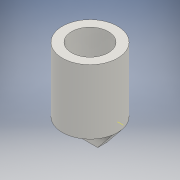
# Autodesk Inventor part: стакан_v2
Saved by Autodesk Inventor 2017.3 (Build 213256000, 256)
## iProperties
Part Number: стакан_v2
Material: Сталь
Document SubType Name: Modeling
Designer: Alexnav
Density: 7.85 g/cm^3
Appearance: По умолчанию
Mass: 1042.58 g
Surface Area: 290.439 cm^2
Volume: 132.812 cm^3
Author: Alexnav
Autodesk Inventor part; units mm, degrees
ref_plane "YZ Plane" through (0, 0, 0) normal (1, 0, 0) x (0, 1, 0)
ref_plane "XZ Plane" through (0, 0, 0) normal (0, 1, 0) x (-1, 0, 0)
ref_plane "XY Plane" through (0, 0, 0) normal (0, 0, 1) x (1, 0, 0)
sketch "Эскиз1" plane through (0, 0, 0) normal (0, 0, 1) x (1, 0, 0)
  circle A0 centre (0, 0) radius 20
  circle A1 centre (0, 0) radius 30
  dimension "d0" = 40
  dimension "d1" = 10
  constraints: 2 centre point, 2 coincident
  measures "d0" diameter of A0
  measures "d1" radial gap between concentric circles of A1 A0
extrude "Выдавливание1" add sketch "Эскиз1" along normal blind 60
sketch "Эскиз2" plane through (0, 0, 0) normal (0, 0, -1) x (-1, 0, 0)
  circle A0 centre (0, 0) radius 30 projected
extrude "Выдавливание2" add sketch "Эскиз2" along normal blind 10
sketch "Эскиз3" plane through (0, 0, -10) normal (0, 0, -1) x (-1, 0, 0)
  circle A0 centre (0, 0) radius 30 projected
  line L0 (-29.5804, 5) -> (29.5804, 5)
  line L1 (29.5804, -5) -> (-29.5804, -5)
  line L2 (42, 0) -> (-42, 0) projected
  dimension "d7" = 10
  constraints: 4 end point, 4 point on circle, 1 horizontal, 1 parallel, 1 other
  measures "d7" distance between parallel lines of L1 L0
extrude "Выдавливание3" add sketch "Эскиз3" along normal blind 20 contours L2 A0 L0 | A0 L1 L2
sketch "Эскиз4" plane through (-29.5804, 5, -10) normal (0, 1, 0) x (1, 0, 0)
  line L0 (59.1608, 0) -> (0, 0) projected
  line L1 (59.1608, 0) -> (59.1608, 20) projected
  line L2 (0, 20) -> (59.1608, 20) projected
  line L3 (0, 0) -> (0, 20) projected
  line L4 (59.1608, 0) -> (59.1608, 20) projected
  line L5 (0, 0) -> (59.1608, 0) projected
  line L6 (0, 0) -> (0, 20) projected
  line L7 (0, 20) -> (59.1608, 20) projected
  circle A0 centre (29.5804, 10) radius 5
  point P0 (29.5804, -10)
  dimension "d11" = 10
  constraints: 1 centre point
  measures "d11" diameter of A0
extrude "Выдавливание4" cut sketch "Эскиз4" along normal through all both and the other way through all contours A0
sketch "Эскиз5" plane through (-29.5804, -5, -10) normal (0, -1, 0) x (1, 0, 0)
  circle A0 centre (29.5804, -10) radius 5 projected
  line L0 (59.1608, -20) -> (0, -20) projected
  line L1 (0, 0) -> (59.1608, 0) projected
  line L2 (0, 0) -> (0, -20) projected
  line L3 (16.199, -20) -> (0, 0)
  line L4 (0, 0) -> (-30.1779, 0)
  line L5 (-30.1779, 0) -> (-30.1779, -20)
  line L6 (-30.1779, -20) -> (16.199, -20)
  line L7 (42.9618, -20) -> (59.1608, 0)
  line L8 (85.3862, 0) -> (85.3862, -20)
  line L9 (85.3862, -20) -> (42.9618, -20)
  line L10 (85.3862, 0) -> (59.1608, 0)
  point P0 (29.5804, 10)
  constraints: 16 end point, 3 perpendicular, 2 point on line, 1 equal length, 1 horizontal, 1 parallel, 1 vertical
extrude "Выдавливание5" cut sketch "Эскиз5" against normal through all contours L0 L7 L10 L8 L9 | L0 L2 L3 | L6 L5 L4 L2
